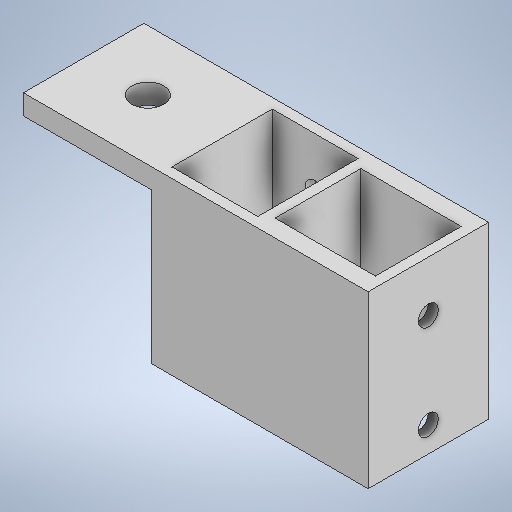
# Autodesk Inventor part: PluckMount
Saved by Autodesk Inventor 2025.1 (Build 291241000, 241)
## iProperties
Created: 2025-12-01
Part Number: PluckMount
Material: Generic
Document SubType Name: Modeling
Designer: Juxin
Density: 1 g/cm^3
Appearance: Default
Author: Juxin
Autodesk Inventor part; units mm, degrees
ref_plane "YZ Plane" through (0, 0, 0) normal (1, 0, 0) x (0, 1, 0)
ref_plane "XZ Plane" through (0, 0, 0) normal (0, 1, 0) x (-1, 0, 0)
ref_plane "XY Plane" through (0, 0, 0) normal (0, 0, 1) x (1, 0, 0)
sketch "Sketch1" plane through (0, 0, 0) normal (0, 1, 0) x (-1, 0, 0)
  line L0 (0, 0) -> (13.589, 0)
  line L1 (13.589, 0) -> (13.589, -15.875)
  line L2 (13.589, -15.875) -> (0, -15.875)
  line L3 (0, -15.875) -> (0, 0)
  line L4 (0, 0) -> (0, -1.143)
  line L5 (0, -1.143) -> (-1.5875, -1.143)
  line L6 (-1.5875, -1.143) -> (-17.4625, -1.143)
  line L7 (-17.4625, -1.143) -> (-17.4625, -14.732)
  line L8 (-17.4625, -14.732) -> (-1.5875, -14.732)
  line L9 (-1.5875, -14.732) -> (-1.5875, -1.143)
  line L10 (13.589, 0) -> (13.589, 1.5875)
  line L11 (13.589, 1.5875) -> (15.1765, 1.5875)
  line L12 (-17.4625, -1.143) -> (-19.05, -1.143)
  line L13 (13.589, -15.875) -> (13.589, -17.4625)
  line L14 (13.589, -17.4625) -> (15.1765, -17.4625)
  line L15 (15.1765, -17.4625) -> (-19.05, -17.4625)
  line L16 (-19.05, -17.4625) -> (-19.05, 1.5875)
  line L17 (-19.05, 1.5875) -> (15.1765, 1.5875)
  line L18 (15.1765, 1.5875) -> (15.1765, -17.4625)
  dimension "d0" = 13.589
  dimension "d1" = 15.875
  dimension "d2" = 1.143
  dimension "d3" = 1.5875
  dimension "d4" = 15.875
  dimension "d5" = 13.589
  dimension "d6" = 1.5875
  dimension "d7" = 1.5875
  dimension "d8" = 1.5875
  dimension "d9" = 1.5875
  dimension "d10" = 1.5875
  constraints: 38 end point, 6 parallel, 5 perpendicular, 4 horizontal, 3 point on line, 1 vertical
  measures "d0" distance of L1.end L2.end
  measures "d1" distance of L0.end L1.end
  measures "d2" distance of L0.start L4.end
  measures "d3" distance of L4.end L5.end
  measures "d4" distance of L8.end L7.end
  measures "d5" distance of L7.end L6.end
  measures "d6" distance of L0.end L10.end
  measures "d7" distance of L10.end L11.end
  measures "d8" distance of L6.end L12.end
  measures "d9" distance of L1.end L13.end
  measures "d10" distance of L13.end L14.end
extrude "Extrusion1" add sketch "Sketch1" along normal blind 25.4 contours L3 L5 L6 L12 L16 L17 L10 L0 | L10 L11 L18 L14 L13 L1 | L3 L2 L13 L15 L16 L12 L7 L8 L9 L5
sketch "Sketch2" plane through (19.05, 0, 1.5875) normal (1, 0, 0) x (0, 0, -1)
  line L0 (16.3195, 25.4) -> (2.7305, 25.4) projected
  line L1 (9.525, 25.4) -> (9.525, 17.399)
  circle A0 centre (9.525, 17.399) radius 1.5875
  line L2 (9.525, 17.399) -> (9.525, 2.413)
  circle A1 centre (9.525, 2.413) radius 1.5875
  point P0 (1.5875, 0)
  dimension "d13" = 8.001
  dimension "d14" = 3.175
  dimension "d15" = 14.986
  dimension "d16" = 3.175
  constraints: 4 end point, 2 centre point, 2 coincident, 2 vertical, 1 midpoint
  measures "d13" distance of L1.start L1.end
  measures "d14" diameter of A0
  measures "d15" distance of L2.start L2.end
  measures "d16" diameter of A1
extrude "Extrusion2" cut sketch "Sketch2" against normal blind 9.525
sketch "Sketch3" plane through (19.05, 0, -17.4625) normal (0, 0, -1) x (-1, 0, 0)
  line L0 (32.639, 0) -> (32.639, 25.4) projected
  line L1 (19.05, 0) -> (19.05, 25.4) projected
  line L2 (32.639, 25.4) -> (19.05, 25.4)
  line L3 (25.8445, 25.4) -> (25.8445, 17.399)
  circle A0 centre (25.8445, 17.399) radius 1.5875
  line L4 (25.8445, 17.399) -> (25.8445, 2.413)
  circle A1 centre (25.8445, 2.413) radius 1.5875
  dimension "d19" = 8.001
  dimension "d20" = 3.175
  dimension "d21" = 14.986
  dimension "d22" = 3.175
  constraints: 6 end point, 2 centre point, 2 coincident, 2 vertical, 1 midpoint, 1 perpendicular
  measures "d19" distance of L3.start L3.end
  measures "d20" diameter of A0
  measures "d21" distance of L4.start L4.end
  measures "d22" diameter of A1
extrude "Extrusion3" cut sketch "Sketch3" against normal blind 9.525
move faces "Move1" translate (0, -1.5875, 0) faces at (1.2912, 0, 1.0583)
sketch "Sketch4" plane through (-15.1765, 25.4, -17.4625) normal (-1, 0, 0) x (0, 0, 1)
  line L0 (0, 0) -> (19.05, 0) projected
  line L1 (0, -26.9875) -> (0, 0) projected
  line L2 (19.05, 0) -> (0, 0)
  line L3 (0, 0) -> (0, -3.175)
  line L4 (0, -3.175) -> (19.05, -3.175)
  line L5 (19.05, -3.175) -> (19.05, 0)
  point P0 (17.4625, -25.4)
  dimension "d28" = 3.175
  constraints: 8 end point, 2 parallel, 1 horizontal, 1 perpendicular, 1 point on line
  measures "d28" distance of L3.end L2.end
extrude "Extrusion4" add sketch "Sketch4" along normal blind 20.32
sketch "Sketch5" plane through (-15.1765, 22.225, -17.4625) normal (0, -1, 0) x (1, 0, 0)
  line L0 (-20.32, 19.05) -> (-20.32, 0) projected
  line L1 (-20.32, 9.525) -> (0, 9.525)
  line L2 (0, 0) -> (0, 19.05) projected
  circle A0 centre (-10.16, 9.525) radius 2.54
  point P0 (15.1765, 17.4625)
  dimension "d31" = 5.08
  constraints: 3 midpoint, 2 end point, 1 centre point
  measures "d31" diameter of A0
extrude "Extrusion5" cut sketch "Sketch5" against normal blind 20.32
body "Solid1"
